Autodesk Fusion 360 part; units mm, degrees
(part 5 of 10)
extrude "Pan blank''''''" add sketch "草图1 (37)" along normal blind 20 separate body makes body 37 in component "Tower_Integrated"
fillet "Outside corner rounds''''''" radius 3 4 edges at (50, 140, 135) (230, 140, 135) (230, 50, 135) (50, 50, 135) on bodies 37 in component "Tower_Integrated"
ref_plane "工作平面2" through (53, 0, 0) normal (1, 0, 0) x (0, 1, 0) in component "Tower_Integrated"
sketch "草图2 (37)" plane through (53, 0, 0) normal (1, 0, 0) x (0, 0, -1) in component "Tower_Integrated"
  line L0 (-135.8318, 53) -> (-129.958, 137)
  line L1 (-129.958, 137) -> (-146, 137)
  line L2 (-146, 137) -> (-146, 53)
  line L3 (-146, 53) -> (-135.8318, 53)
  dimension "d1948" = 135.8318
  dimension "d1950" = 129.958
  dimension "d1952" = 146
  constraint horizontal L1
  constraint vertical L2
  constraint horizontal L3
  measures "d1948" horizontal distance of origin L0.start
  measures "d1950" horizontal distance of origin L0.end
  measures "d1952" horizontal distance of origin L1.end
extrude "Sloped catch cavity''''''" cut sketch "草图2 (37)" along normal blind 174 bodies 37 in component "Tower_Integrated"
ref_plane "工作平面3" through (178, 0, 0) normal (1, 0, 0) x (0, 1, 0) in component "Tower_Integrated"
sketch "草图3 (13)" plane through (178, 0, 0) normal (1, 0, 0) x (0, 0, -1) in component "Tower_Integrated"
  line L0 (-125, 137) -> (-125, 165)
  line L1 (-125, 165) -> (-128, 165)
  line L2 (-128, 165) -> (-129.958, 137)
  line L3 (-129.958, 137) -> (-125, 137)
  dimension "d1960" = 128
  dimension "d1961" = 129.958
  constraint vertical L0
  constraint horizontal L1
  constraint horizontal L3
  measures "d1960" horizontal distance of origin L1.end
  measures "d1961" horizontal distance of origin L2.end
extrude "Drain tongue floor''''''" add sketch "草图3 (13)" along normal blind 34 bodies 37 in component "Tower_Integrated"
ref_plane "工作平面4" through (178, 0, 0) normal (1, 0, 0) x (0, 1, 0) in component "Tower_Integrated"
sketch "草图4 (13)" plane through (178, 0, 0) normal (1, 0, 0) x (0, 0, -1) in component "Tower_Integrated"
  line L0 (-125, 137) -> (-125, 165)
  line L1 (-125, 165) -> (-134, 165)
  line L2 (-134, 165) -> (-135.958, 137)
  line L3 (-135.958, 137) -> (-125, 137)
  dimension "d1969" = 134
  dimension "d1970" = 135.958
  constraint vertical L0
  constraint horizontal L1
  constraint horizontal L3
  measures "d1969" horizontal distance of origin L1.end
  measures "d1970" horizontal distance of origin L2.end
extrude "Tongue side rail''''''" add sketch "草图4 (13)" along normal blind 3 bodies 37 in component "Tower_Integrated"
ref_plane "工作平面5" through (209, 0, 0) normal (1, 0, 0) x (0, 1, 0) in component "Tower_Integrated"
sketch "草图5 (13)" plane through (209, 0, 0) normal (1, 0, 0) x (0, 0, -1) in component "Tower_Integrated"
  line L0 (-125, 137) -> (-125, 165)
  line L1 (-125, 165) -> (-134, 165)
  line L2 (-134, 165) -> (-135.958, 137)
  line L3 (-135.958, 137) -> (-125, 137)
  dimension "d1978" = 134
  dimension "d1979" = 135.958
  constraint vertical L0
  constraint horizontal L1
  constraint horizontal L3
  measures "d1978" horizontal distance of origin L1.end
  measures "d1979" horizontal distance of origin L2.end
extrude "Tongue side rail (1)''''''" add sketch "草图5 (13)" along normal blind 3 bodies 37 in component "Tower_Integrated"
ref_plane "工作平面6" through (181, 0, 0) normal (1, 0, 0) x (0, 1, 0) in component "Tower_Integrated"
sketch "草图6 (13)" plane through (181, 0, 0) normal (1, 0, 0) x (0, 0, -1) in component "Tower_Integrated"
  line L0 (-129.958, 137) -> (-128, 165)
  line L1 (-128, 165) -> (-146, 165)
  line L2 (-146, 165) -> (-146, 137)
  line L3 (-146, 137) -> (-129.958, 137)
  dimension "d1984" = 129.958
  dimension "d1986" = 128
  dimension "d1988" = 146
  constraint horizontal L1
  constraint vertical L2
  constraint horizontal L3
  measures "d1984" horizontal distance of origin L0.start
  measures "d1986" horizontal distance of origin L0.end
  measures "d1988" horizontal distance of origin L1.end
extrude "Open drain mouth''''''" cut sketch "草图6 (13)" along normal blind 28 bodies 37 in component "Tower_Integrated"
ref_plane "工作平面7" through (0, 0, 125) normal (0, 0, 1) x (1, 0, 0) in component "Tower_Integrated"
sketch "草图7 (13)" plane through (0, 0, 125) normal (0, 0, 1) x (1, 0, 0) in component "Tower_Integrated"
  line L0 (53, 53) -> (65, 53)
  line L1 (65, 53) -> (65, 65)
  line L2 (65, 65) -> (53, 65)
  line L3 (53, 65) -> (53, 53)
  dimension "d1995" = 12
  dimension "d1996" = 12
  constraint horizontal L0
  constraint vertical L1
  constraint horizontal L2
  constraint vertical L3
  measures "d1995" horizontal distance of L0.start L0.end
  measures "d1996" vertical distance of L0.end L1.end
extrude "Grate seat 00''''''" add sketch "草图7 (13)" along normal blind 16 bodies 37 in component "Tower_Integrated"
ref_plane "工作平面8" through (0, 0, 125) normal (0, 0, 1) x (1, 0, 0) in component "Tower_Integrated"
sketch "草图8 (13)" plane through (0, 0, 125) normal (0, 0, 1) x (1, 0, 0) in component "Tower_Integrated"
  line L0 (53, 125) -> (65, 125)
  line L1 (65, 125) -> (65, 137)
  line L2 (65, 137) -> (53, 137)
  line L3 (53, 137) -> (53, 125)
  dimension "d2002" = 125
  dimension "d2003" = 12
  dimension "d2004" = 12
  constraint horizontal L0
  constraint vertical L1
  constraint horizontal L2
  constraint vertical L3
  measures "d2002" vertical distance of origin L0.start
  measures "d2003" horizontal distance of L0.start L0.end
  measures "d2004" vertical distance of L0.end L1.end
extrude "Grate seat 01''''''" add sketch "草图8 (13)" along normal blind 16 bodies 37 in component "Tower_Integrated"
ref_plane "工作平面9" through (0, 0, 125) normal (0, 0, 1) x (1, 0, 0) in component "Tower_Integrated"
sketch "草图9 (13)" plane through (0, 0, 125) normal (0, 0, 1) x (1, 0, 0) in component "Tower_Integrated"
  line L0 (215, 53) -> (227, 53)
  line L1 (227, 53) -> (227, 65)
  line L2 (227, 65) -> (215, 65)
  line L3 (215, 65) -> (215, 53)
  dimension "d2009" = 215
  dimension "d2011" = 12
  dimension "d2012" = 12
  constraint horizontal L0
  constraint vertical L1
  constraint horizontal L2
  constraint vertical L3
  measures "d2009" horizontal distance of origin L0.start
  measures "d2011" horizontal distance of L0.start L0.end
  measures "d2012" vertical distance of L0.end L1.end
extrude "Grate seat 10''''''" add sketch "草图9 (13)" along normal blind 16 bodies 37 in component "Tower_Integrated"
ref_plane "工作平面10" through (0, 0, 125) normal (0, 0, 1) x (1, 0, 0) in component "Tower_Integrated"
sketch "草图10 (13)" plane through (0, 0, 125) normal (0, 0, 1) x (1, 0, 0) in component "Tower_Integrated"
  line L0 (215, 125) -> (227, 125)
  line L1 (227, 125) -> (227, 137)
  line L2 (227, 137) -> (215, 137)
  line L3 (215, 137) -> (215, 125)
  dimension "d2017" = 215
  dimension "d2018" = 125
  dimension "d2019" = 12
  dimension "d2020" = 12
  constraint horizontal L0
  constraint vertical L1
  constraint horizontal L2
  constraint vertical L3
  measures "d2017" horizontal distance of origin L0.start
  measures "d2018" vertical distance of origin L0.start
  measures "d2019" horizontal distance of L0.start L0.end
  measures "d2020" vertical distance of L0.end L1.end
extrude "Grate seat 11''''''" add sketch "草图10 (13)" along normal blind 16 bodies 37 in component "Tower_Integrated"
ref_plane "工作平面11" through (178, 0, 0) normal (1, 0, 0) x (0, 1, 0) in component "Tower_Integrated"
sketch "草图11 (13)" plane through (178, 0, 0) normal (1, 0, 0) x (0, 0, -1) in component "Tower_Integrated"
  line L0 (-124.8, 163) -> (-124.8, 164)
  line L1 (-124.8, 164) -> (-125.6, 164)
  line L2 (-125.6, 164) -> (-125.6, 163)
  line L3 (-125.6, 163) -> (-124.8, 163)
  dimension "d2025" = 124.8
  dimension "d2026" = 163
  dimension "d2027" = 164
  dimension "d2028" = 125.6
  constraint vertical L0
  constraint horizontal L1
  constraint vertical L2
  constraint horizontal L3
  measures "d2025" horizontal distance of origin L0.start
  measures "d2026" vertical distance of origin L0.start
  measures "d2027" vertical distance of origin L0.end
  measures "d2028" horizontal distance of origin L1.end
extrude "Drip break underside groove''''''" cut sketch "草图11 (13)" along normal blind 34 bodies 37 in component "Tower_Integrated"
ref_plane "工作平面1" through (0, 0, 141) normal (0, 0, 1) x (1, 0, 0) in component "UP_RemovableGrate"
sketch "草图1 (38)" plane through (0, 0, 141) normal (0, 0, 1) x (1, 0, 0) in component "UP_RemovableGrate"
  line L0 (53.3, 53.3) -> (226.7, 53.3)
  line L1 (226.7, 53.3) -> (226.7, 136.7)
  line L2 (226.7, 136.7) -> (53.3, 136.7)
  line L3 (53.3, 136.7) -> (53.3, 53.3)
  dimension "d2035" = 173.4
  dimension "d2036" = 83.4
  constraint horizontal L0
  constraint vertical L1
  constraint horizontal L2
  constraint vertical L3
  measures "d2035" horizontal distance of L0.start L0.end
  measures "d2036" vertical distance of L0.end L1.end
extrude "Horizontal removable deck''''''" add sketch "草图1 (38)" along normal blind 4 separate body makes body 38 in component "UP_RemovableGrate"
ref_plane "工作平面2" through (0, 0, 141) normal (0, 0, 1) x (1, 0, 0) in component "UP_RemovableGrate"
sketch "草图2 (38)" plane through (0, 0, 141) normal (0, 0, 1) x (1, 0, 0) in component "UP_RemovableGrate"
  line L0 (68, 60.3) -> (72, 60.3)
  line L1 (72, 60.3) -> (72, 129.7)
  line L2 (72, 129.7) -> (68, 129.7)
  line L3 (68, 129.7) -> (68, 60.3)
  dimension "d2041" = 68
  dimension "d2043" = 4
  dimension "d2044" = 69.4
  constraint horizontal L0
  constraint vertical L1
  constraint horizontal L2
  constraint vertical L3
  measures "d2041" horizontal distance of origin L0.start
  measures "d2043" horizontal distance of L0.start L0.end
  measures "d2044" vertical distance of L0.end L1.end
extrude "Drain slot 1''''''" cut sketch "草图2 (38)" along normal blind 4 bodies 38 in component "UP_RemovableGrate"
ref_plane "工作平面3" through (0, 0, 141) normal (0, 0, 1) x (1, 0, 0) in component "UP_RemovableGrate"
sketch "草图3 (14)" plane through (0, 0, 141) normal (0, 0, 1) x (1, 0, 0) in component "UP_RemovableGrate"
  line L0 (78, 60.3) -> (82, 60.3)
  line L1 (82, 60.3) -> (82, 129.7)
  line L2 (82, 129.7) -> (78, 129.7)
  line L3 (78, 129.7) -> (78, 60.3)
  dimension "d2049" = 78
  dimension "d2051" = 4
  dimension "d2052" = 69.4
  constraint horizontal L0
  constraint vertical L1
  constraint horizontal L2
  constraint vertical L3
  measures "d2049" horizontal distance of origin L0.start
  measures "d2051" horizontal distance of L0.start L0.end
  measures "d2052" vertical distance of L0.end L1.end
extrude "Drain slot 2''''''" cut sketch "草图3 (14)" along normal blind 4 bodies 38 in component "UP_RemovableGrate"
ref_plane "工作平面4" through (0, 0, 141) normal (0, 0, 1) x (1, 0, 0) in component "UP_RemovableGrate"
sketch "草图4 (14)" plane through (0, 0, 141) normal (0, 0, 1) x (1, 0, 0) in component "UP_RemovableGrate"
  line L0 (88, 60.3) -> (92, 60.3)
  line L1 (92, 60.3) -> (92, 129.7)
  line L2 (92, 129.7) -> (88, 129.7)
  line L3 (88, 129.7) -> (88, 60.3)
  dimension "d2057" = 88
  dimension "d2059" = 4
  dimension "d2060" = 69.4
  constraint horizontal L0
  constraint vertical L1
  constraint horizontal L2
  constraint vertical L3
  measures "d2057" horizontal distance of origin L0.start
  measures "d2059" horizontal distance of L0.start L0.end
  measures "d2060" vertical distance of L0.end L1.end
extrude "Drain slot 3''''''" cut sketch "草图4 (14)" along normal blind 4 bodies 38 in component "UP_RemovableGrate"
ref_plane "工作平面5" through (0, 0, 141) normal (0, 0, 1) x (1, 0, 0) in component "UP_RemovableGrate"
sketch "草图5 (14)" plane through (0, 0, 141) normal (0, 0, 1) x (1, 0, 0) in component "UP_RemovableGrate"
  line L0 (98, 60.3) -> (102, 60.3)
  line L1 (102, 60.3) -> (102, 129.7)
  line L2 (102, 129.7) -> (98, 129.7)
  line L3 (98, 129.7) -> (98, 60.3)
  dimension "d2065" = 98
  dimension "d2067" = 4
  dimension "d2068" = 69.4
  constraint horizontal L0
  constraint vertical L1
  constraint horizontal L2
  constraint vertical L3
  measures "d2065" horizontal distance of origin L0.start
  measures "d2067" horizontal distance of L0.start L0.end
  measures "d2068" vertical distance of L0.end L1.end
extrude "Drain slot 4''''''" cut sketch "草图5 (14)" along normal blind 4 bodies 38 in component "UP_RemovableGrate"
ref_plane "工作平面6" through (0, 0, 141) normal (0, 0, 1) x (1, 0, 0) in component "UP_RemovableGrate"
sketch "草图6 (14)" plane through (0, 0, 141) normal (0, 0, 1) x (1, 0, 0) in component "UP_RemovableGrate"
  line L0 (108, 60.3) -> (112, 60.3)
  line L1 (112, 60.3) -> (112, 129.7)
  line L2 (112, 129.7) -> (108, 129.7)
  line L3 (108, 129.7) -> (108, 60.3)
  dimension "d2073" = 108
  dimension "d2075" = 4
  dimension "d2076" = 69.4
  constraint horizontal L0
  constraint vertical L1
  constraint horizontal L2
  constraint vertical L3
  measures "d2073" horizontal distance of origin L0.start
  measures "d2075" horizontal distance of L0.start L0.end
  measures "d2076" vertical distance of L0.end L1.end
extrude "Drain slot 5''''''" cut sketch "草图6 (14)" along normal blind 4 bodies 38 in component "UP_RemovableGrate"
ref_plane "工作平面7" through (0, 0, 141) normal (0, 0, 1) x (1, 0, 0) in component "UP_RemovableGrate"
sketch "草图7 (14)" plane through (0, 0, 141) normal (0, 0, 1) x (1, 0, 0) in component "UP_RemovableGrate"
  line L0 (118, 60.3) -> (122, 60.3)
  line L1 (122, 60.3) -> (122, 129.7)
  line L2 (122, 129.7) -> (118, 129.7)
  line L3 (118, 129.7) -> (118, 60.3)
  dimension "d2081" = 118
  dimension "d2083" = 4
  dimension "d2084" = 69.4
  constraint horizontal L0
  constraint vertical L1
  constraint horizontal L2
  constraint vertical L3
  measures "d2081" horizontal distance of origin L0.start
  measures "d2083" horizontal distance of L0.start L0.end
  measures "d2084" vertical distance of L0.end L1.end
extrude "Drain slot 6''''''" cut sketch "草图7 (14)" along normal blind 4 bodies 38 in component "UP_RemovableGrate"
ref_plane "工作平面8" through (0, 0, 141) normal (0, 0, 1) x (1, 0, 0) in component "UP_RemovableGrate"
sketch "草图8 (14)" plane through (0, 0, 141) normal (0, 0, 1) x (1, 0, 0) in component "UP_RemovableGrate"
  line L0 (128, 60.3) -> (132, 60.3)
  line L1 (132, 60.3) -> (132, 129.7)
  line L2 (132, 129.7) -> (128, 129.7)
  line L3 (128, 129.7) -> (128, 60.3)
  dimension "d2089" = 128
  dimension "d2091" = 4
  dimension "d2092" = 69.4
  constraint horizontal L0
  constraint vertical L1
  constraint horizontal L2
  constraint vertical L3
  measures "d2089" horizontal distance of origin L0.start
  measures "d2091" horizontal distance of L0.start L0.end
  measures "d2092" vertical distance of L0.end L1.end
extrude "Drain slot 7''''''" cut sketch "草图8 (14)" along normal blind 4 bodies 38 in component "UP_RemovableGrate"
ref_plane "工作平面9" through (0, 0, 141) normal (0, 0, 1) x (1, 0, 0) in component "UP_RemovableGrate"
sketch "草图9 (14)" plane through (0, 0, 141) normal (0, 0, 1) x (1, 0, 0) in component "UP_RemovableGrate"
  line L0 (138, 60.3) -> (142, 60.3)
  line L1 (142, 60.3) -> (142, 129.7)
  line L2 (142, 129.7) -> (138, 129.7)
  line L3 (138, 129.7) -> (138, 60.3)
  dimension "d2097" = 138
  dimension "d2099" = 4
  dimension "d2100" = 69.4
  constraint horizontal L0
  constraint vertical L1
  constraint horizontal L2
  constraint vertical L3
  measures "d2097" horizontal distance of origin L0.start
  measures "d2099" horizontal distance of L0.start L0.end
  measures "d2100" vertical distance of L0.end L1.end
extrude "Drain slot 8''''''" cut sketch "草图9 (14)" along normal blind 4 bodies 38 in component "UP_RemovableGrate"
ref_plane "工作平面10" through (0, 0, 141) normal (0, 0, 1) x (1, 0, 0) in component "UP_RemovableGrate"
sketch "草图10 (14)" plane through (0, 0, 141) normal (0, 0, 1) x (1, 0, 0) in component "UP_RemovableGrate"
  line L0 (148, 60.3) -> (152, 60.3)
  line L1 (152, 60.3) -> (152, 129.7)
  line L2 (152, 129.7) -> (148, 129.7)
  line L3 (148, 129.7) -> (148, 60.3)
  dimension "d2105" = 148
  dimension "d2107" = 4
  dimension "d2108" = 69.4
  constraint horizontal L0
  constraint vertical L1
  constraint horizontal L2
  constraint vertical L3
  measures "d2105" horizontal distance of origin L0.start
  measures "d2107" horizontal distance of L0.start L0.end
  measures "d2108" vertical distance of L0.end L1.end
extrude "Drain slot 9''''''" cut sketch "草图10 (14)" along normal blind 4 bodies 38 in component "UP_RemovableGrate"
ref_plane "工作平面11" through (0, 0, 141) normal (0, 0, 1) x (1, 0, 0) in component "UP_RemovableGrate"
sketch "草图11 (14)" plane through (0, 0, 141) normal (0, 0, 1) x (1, 0, 0) in component "UP_RemovableGrate"
  line L0 (158, 60.3) -> (162, 60.3)
  line L1 (162, 60.3) -> (162, 129.7)
  line L2 (162, 129.7) -> (158, 129.7)
  line L3 (158, 129.7) -> (158, 60.3)
  dimension "d2113" = 158
  dimension "d2115" = 4
  dimension "d2116" = 69.4
  constraint horizontal L0
  constraint vertical L1
  constraint horizontal L2
  constraint vertical L3
  measures "d2113" horizontal distance of origin L0.start
  measures "d2115" horizontal distance of L0.start L0.end
  measures "d2116" vertical distance of L0.end L1.end
extrude "Drain slot 10''''''" cut sketch "草图11 (14)" along normal blind 4 bodies 38 in component "UP_RemovableGrate"
ref_plane "工作平面12" through (0, 0, 141) normal (0, 0, 1) x (1, 0, 0) in component "UP_RemovableGrate"
sketch "草图12 (13)" plane through (0, 0, 141) normal (0, 0, 1) x (1, 0, 0) in component "UP_RemovableGrate"
  line L0 (168, 60.3) -> (172, 60.3)
  line L1 (172, 60.3) -> (172, 129.7)
  line L2 (172, 129.7) -> (168, 129.7)
  line L3 (168, 129.7) -> (168, 60.3)
  dimension "d2121" = 168
  dimension "d2123" = 4
  dimension "d2124" = 69.4
  constraint horizontal L0
  constraint vertical L1
  constraint horizontal L2
  constraint vertical L3
  measures "d2121" horizontal distance of origin L0.start
  measures "d2123" horizontal distance of L0.start L0.end
  measures "d2124" vertical distance of L0.end L1.end
extrude "Drain slot 11''''''" cut sketch "草图12 (13)" along normal blind 4 bodies 38 in component "UP_RemovableGrate"
ref_plane "工作平面13" through (0, 0, 141) normal (0, 0, 1) x (1, 0, 0) in component "UP_RemovableGrate"
sketch "草图13 (13)" plane through (0, 0, 141) normal (0, 0, 1) x (1, 0, 0) in component "UP_RemovableGrate"
  line L0 (178, 60.3) -> (182, 60.3)
  line L1 (182, 60.3) -> (182, 129.7)
  line L2 (182, 129.7) -> (178, 129.7)
  line L3 (178, 129.7) -> (178, 60.3)
  dimension "d2129" = 178
  dimension "d2131" = 4
  dimension "d2132" = 69.4
  constraint horizontal L0
  constraint vertical L1
  constraint horizontal L2
  constraint vertical L3
  measures "d2129" horizontal distance of origin L0.start
  measures "d2131" horizontal distance of L0.start L0.end
  measures "d2132" vertical distance of L0.end L1.end
extrude "Drain slot 12''''" cut sketch "草图13 (13)" along normal blind 4 bodies 38 in component "UP_RemovableGrate"
ref_plane "工作平面14" through (0, 0, 141) normal (0, 0, 1) x (1, 0, 0) in component "UP_RemovableGrate"
sketch "草图14 (11)" plane through (0, 0, 141) normal (0, 0, 1) x (1, 0, 0) in component "UP_RemovableGrate"
  line L0 (188, 60.3) -> (192, 60.3)
  line L1 (192, 60.3) -> (192, 129.7)
  line L2 (192, 129.7) -> (188, 129.7)
  line L3 (188, 129.7) -> (188, 60.3)
  dimension "d2137" = 188
  dimension "d2139" = 4
  dimension "d2140" = 69.4
  constraint horizontal L0
  constraint vertical L1
  constraint horizontal L2
  constraint vertical L3
  measures "d2137" horizontal distance of origin L0.start
  measures "d2139" horizontal distance of L0.start L0.end
  measures "d2140" vertical distance of L0.end L1.end
extrude "Drain slot 13''''" cut sketch "草图14 (11)" along normal blind 4 bodies 38 in component "UP_RemovableGrate"
ref_plane "工作平面15" through (0, 0, 141) normal (0, 0, 1) x (1, 0, 0) in component "UP_RemovableGrate"
sketch "草图15 (11)" plane through (0, 0, 141) normal (0, 0, 1) x (1, 0, 0) in component "UP_RemovableGrate"
  line L0 (198, 60.3) -> (202, 60.3)
  line L1 (202, 60.3) -> (202, 129.7)
  line L2 (202, 129.7) -> (198, 129.7)
  line L3 (198, 129.7) -> (198, 60.3)
  dimension "d2145" = 198
  dimension "d2147" = 4
  dimension "d2148" = 69.4
  constraint horizontal L0
  constraint vertical L1
  constraint horizontal L2
  constraint vertical L3
  measures "d2145" horizontal distance of origin L0.start
  measures "d2147" horizontal distance of L0.start L0.end
  measures "d2148" vertical distance of L0.end L1.end
extrude "Drain slot 14'''" cut sketch "草图15 (11)" along normal blind 4 bodies 38 in component "UP_RemovableGrate"
ref_plane "工作平面16" through (0, 0, 141) normal (0, 0, 1) x (1, 0, 0) in component "UP_RemovableGrate"
sketch "草图16 (4)" plane through (0, 0, 141) normal (0, 0, 1) x (1, 0, 0) in component "UP_RemovableGrate"
  line L0 (208, 60.3) -> (212, 60.3)
  line L1 (212, 60.3) -> (212, 129.7)
  line L2 (212, 129.7) -> (208, 129.7)
  line L3 (208, 129.7) -> (208, 60.3)
  dimension "d2153" = 208
  dimension "d2155" = 4
  dimension "d2156" = 69.4
  constraint horizontal L0
  constraint vertical L1
  constraint horizontal L2
  constraint vertical L3
  measures "d2153" horizontal distance of origin L0.start
  measures "d2155" horizontal distance of L0.start L0.end
  measures "d2156" vertical distance of L0.end L1.end
extrude "Drain slot 15'''" cut sketch "草图16 (4)" along normal blind 4 bodies 38 in component "UP_RemovableGrate"
ref_plane "工作平面17" through (0, 0, 141) normal (0, 0, 1) x (1, 0, 0) in component "UP_RemovableGrate"
sketch "草图17 (4)" plane through (0, 0, 141) normal (0, 0, 1) x (1, 0, 0) in component "UP_RemovableGrate"
  line L0 (132, 132.7) -> (148, 132.7)
  line L1 (148, 132.7) -> (148, 137.7)
  line L2 (148, 137.7) -> (132, 137.7)
  line L3 (132, 137.7) -> (132, 132.7)
  dimension "d2161" = 132
  dimension "d2162" = 132.7
  dimension "d2163" = 16
  dimension "d2164" = 5
  constraint horizontal L0
  constraint vertical L1
  constraint horizontal L2
  constraint vertical L3
  measures "d2161" horizontal distance of origin L0.start
  measures "d2162" vertical distance of origin L0.start
  measures "d2163" horizontal distance of L0.start L0.end
  measures "d2164" vertical distance of L0.end L1.end
extrude "Finger lift notch''''''" cut sketch "草图17 (4)" along normal blind 4 bodies 38 in component "UP_RemovableGrate"
ref_plane "工作平面1" through (0, 0, 0) normal (0, 0, 1) x (1, 0, 0) in component "Tower_SideFrame_1"
sketch "草图1 (39)" plane through (0, 0, 0) normal (0, 0, 1) x (1, 0, 0) in component "Tower_SideFrame_1"
  line L0 (50, 50) -> (58, 50)
  line L1 (58, 50) -> (58, 140)
  line L2 (58, 140) -> (50, 140)
  line L3 (50, 140) -> (50, 50)
  dimension "d2169" = 50
  dimension "d2170" = 50
  dimension "d2171" = 8
  dimension "d2172" = 90
  constraint horizontal L0
  constraint vertical L1
  constraint horizontal L2
  constraint vertical L3
  measures "d2169" horizontal distance of origin L0.start
  measures "d2170" vertical distance of origin L0.start
  measures "d2171" horizontal distance of L0.start L0.end
  measures "d2172" vertical distance of L0.end L1.end
extrude "Portal frame blank" add sketch "草图1 (39)" along normal blind 125 separate body makes body 39 in component "Tower_SideFrame_1"
ref_plane "工作平面2" through (50, 0, 0) normal (1, 0, 0) x (0, 1, 0) in component "Tower_SideFrame_1"
sketch "草图2 (39)" plane through (50, 0, 0) normal (1, 0, 0) x (0, 0, -1) in component "Tower_SideFrame_1"
  line L0 (-8, 62) -> (-8, 128)
  line L1 (-8, 128) -> (-117, 128)
  line L2 (-117, 128) -> (-117, 62)
  line L3 (-117, 62) -> (-8, 62)
  dimension "d2177" = 8
  dimension "d2178" = 62
  dimension "d2179" = 128
  dimension "d2180" = 117
  constraint vertical L0
  constraint horizontal L1
  constraint vertical L2
  constraint horizontal L3
  measures "d2177" horizontal distance of origin L0.start
  measures "d2178" vertical distance of origin L0.start
  measures "d2179" vertical distance of origin L0.end
  measures "d2180" horizontal distance of origin L1.end
extrude "Open portal" cut sketch "草图2 (39)" along normal blind 8 bodies 39 in component "Tower_SideFrame_1"
ref_plane "工作平面3" through (0, 0, 125) normal (0, 0, 1) x (1, 0, 0) in component "Tower_SideFrame_1"
sketch "草图3 (15)" plane through (0, 0, 125) normal (0, 0, 1) x (1, 0, 0) in component "Tower_SideFrame_1"
  line L0 (51.5, 55.5) -> (56.5, 55.5)
  line L1 (56.5, 55.5) -> (56.5, 60.5)
  line L2 (56.5, 60.5) -> (51.5, 60.5)
  line L3 (51.5, 60.5) -> (51.5, 55.5)
  dimension "d2185" = 51.5
  dimension "d2186" = 55.5
  dimension "d2187" = 5
  dimension "d2188" = 5
  constraint horizontal L0
  constraint vertical L1
  constraint horizontal L2
  constraint vertical L3
  measures "d2185" horizontal distance of origin L0.start
  measures "d2186" vertical distance of origin L0.start
  measures "d2187" horizontal distance of L0.start L0.end
  measures "d2188" vertical distance of L0.end L1.end
extrude "Upper tray locating key" add sketch "草图3 (15)" along normal blind 1.5 bodies 39 in component "Tower_SideFrame_1"
ref_plane "工作平面4" through (0, 0, 125) normal (0, 0, 1) x (1, 0, 0) in component "Tower_SideFrame_1"
sketch "草图4 (15)" plane through (0, 0, 125) normal (0, 0, 1) x (1, 0, 0) in component "Tower_SideFrame_1"
  line L0 (51.5, 129.5) -> (56.5, 129.5)
  line L1 (56.5, 129.5) -> (56.5, 134.5)
  line L2 (56.5, 134.5) -> (51.5, 134.5)
  line L3 (51.5, 134.5) -> (51.5, 129.5)
  dimension "d2193" = 51.5
  dimension "d2194" = 129.5
  dimension "d2195" = 5
  dimension "d2196" = 5
  constraint horizontal L0
  constraint vertical L1
  constraint horizontal L2
  constraint vertical L3
  measures "d2193" horizontal distance of origin L0.start
  measures "d2194" vertical distance of origin L0.start
  measures "d2195" horizontal distance of L0.start L0.end
  measures "d2196" vertical distance of L0.end L1.end
extrude "Upper tray locating key (1)" add sketch "草图4 (15)" along normal blind 1.5 bodies 39 in component "Tower_SideFrame_1"
ref_plane "工作平面1" through (0, 0, 0) normal (0, 0, 1) x (1, 0, 0) in component "Tower_SideFrame_2"
sketch "草图1 (40)" plane through (0, 0, 0) normal (0, 0, 1) x (1, 0, 0) in component "Tower_SideFrame_2"
  line L0 (222, 50) -> (230, 50)
  line L1 (230, 50) -> (230, 140)
  line L2 (230, 140) -> (222, 140)
  line L3 (222, 140) -> (222, 50)
  dimension "d2201" = 222
  dimension "d2202" = 50
  dimension "d2203" = 8
  dimension "d2204" = 90
  constraint horizontal L0
  constraint vertical L1
  constraint horizontal L2
  constraint vertical L3
  measures "d2201" horizontal distance of origin L0.start
  measures "d2202" vertical distance of origin L0.start
  measures "d2203" horizontal distance of L0.start L0.end
  measures "d2204" vertical distance of L0.end L1.end
extrude "Portal frame blank'" add sketch "草图1 (40)" along normal blind 125 separate body makes body 40 in component "Tower_SideFrame_2"
ref_plane "工作平面2" through (222, 0, 0) normal (1, 0, 0) x (0, 1, 0) in component "Tower_SideFrame_2"
sketch "草图2 (40)" plane through (222, 0, 0) normal (1, 0, 0) x (0, 0, -1) in component "Tower_SideFrame_2"
  line L0 (-8, 62) -> (-8, 128)
  line L1 (-8, 128) -> (-117, 128)
  line L2 (-117, 128) -> (-117, 62)
  line L3 (-117, 62) -> (-8, 62)
  dimension "d2209" = 8
  dimension "d2210" = 62
  dimension "d2211" = 128
  dimension "d2212" = 117
  constraint vertical L0
  constraint horizontal L1
  constraint vertical L2
  constraint horizontal L3
  measures "d2209" horizontal distance of origin L0.start
  measures "d2210" vertical distance of origin L0.start
  measures "d2211" vertical distance of origin L0.end
  measures "d2212" horizontal distance of origin L1.end
extrude "Open portal'" cut sketch "草图2 (40)" along normal blind 8 bodies 40 in component "Tower_SideFrame_2"
ref_plane "工作平面3" through (0, 0, 125) normal (0, 0, 1) x (1, 0, 0) in component "Tower_SideFrame_2"
sketch "草图3 (16)" plane through (0, 0, 125) normal (0, 0, 1) x (1, 0, 0) in component "Tower_SideFrame_2"
  line L0 (223.5, 55.5) -> (228.5, 55.5)
  line L1 (228.5, 55.5) -> (228.5, 60.5)
  line L2 (228.5, 60.5) -> (223.5, 60.5)
  line L3 (223.5, 60.5) -> (223.5, 55.5)
  dimension "d2217" = 223.5
  dimension "d2218" = 55.5
  dimension "d2219" = 5
  dimension "d2220" = 5
  constraint horizontal L0
  constraint vertical L1
  constraint horizontal L2
  constraint vertical L3
  measures "d2217" horizontal distance of origin L0.start
  measures "d2218" vertical distance of origin L0.start
  measures "d2219" horizontal distance of L0.start L0.end
  measures "d2220" vertical distance of L0.end L1.end
extrude "Upper tray locating key'" add sketch "草图3 (16)" along normal blind 1.5 bodies 40 in component "Tower_SideFrame_2"
ref_plane "工作平面4" through (0, 0, 125) normal (0, 0, 1) x (1, 0, 0) in component "Tower_SideFrame_2"
sketch "草图4 (16)" plane through (0, 0, 125) normal (0, 0, 1) x (1, 0, 0) in component "Tower_SideFrame_2"
  line L0 (223.5, 129.5) -> (228.5, 129.5)
  line L1 (228.5, 129.5) -> (228.5, 134.5)
  line L2 (228.5, 134.5) -> (223.5, 134.5)
  line L3 (223.5, 134.5) -> (223.5, 129.5)
  dimension "d2225" = 223.5
  dimension "d2226" = 129.5
  dimension "d2227" = 5
  dimension "d2228" = 5
  constraint horizontal L0
  constraint vertical L1
  constraint horizontal L2
  constraint vertical L3
  measures "d2225" horizontal distance of origin L0.start
  measures "d2226" vertical distance of origin L0.start
  measures "d2227" horizontal distance of L0.start L0.end
  measures "d2228" vertical distance of L0.end L1.end
extrude "Upper tray locating key (1)'" add sketch "草图4 (16)" along normal blind 1.5 bodies 40 in component "Tower_SideFrame_2"
ref_plane "工作平面12" through (0, 0, 125) normal (0, 0, 1) x (1, 0, 0) in component "Tower_Integrated"
sketch "草图12 (14)" plane through (0, 0, 125) normal (0, 0, 1) x (1, 0, 0) in component "Tower_Integrated"
  line L0 (51.25, 55.25) -> (56.75, 55.25)
  line L1 (56.75, 55.25) -> (56.75, 60.75)
  line L2 (56.75, 60.75) -> (51.25, 60.75)
  line L3 (51.25, 60.75) -> (51.25, 55.25)
  dimension "d2233" = 51.25
  dimension "d2234" = 55.25
  dimension "d2235" = 5.5
  dimension "d2236" = 5.5
  constraint horizontal L0
  constraint vertical L1
  constraint horizontal L2
  constraint vertical L3
  measures "d2233" horizontal distance of origin L0.start
  measures "d2234" vertical distance of origin L0.start
  measures "d2235" horizontal distance of L0.start L0.end
  measures "d2236" vertical distance of L0.end L1.end
extrude "Upper frame key socket" cut sketch "草图12 (14)" along normal blind 1.8 bodies 37 in component "Tower_Integrated"
ref_plane "工作平面13" through (0, 0, 125) normal (0, 0, 1) x (1, 0, 0) in component "Tower_Integrated"
sketch "草图13 (14)" plane through (0, 0, 125) normal (0, 0, 1) x (1, 0, 0) in component "Tower_Integrated"
  line L0 (51.25, 129.25) -> (56.75, 129.25)
  line L1 (56.75, 129.25) -> (56.75, 134.75)
  line L2 (56.75, 134.75) -> (51.25, 134.75)
  line L3 (51.25, 134.75) -> (51.25, 129.25)
  dimension "d2241" = 51.25
  dimension "d2242" = 129.25
  dimension "d2243" = 5.5
  dimension "d2244" = 5.5
  constraint horizontal L0
  constraint vertical L1
  constraint horizontal L2
  constraint vertical L3
  measures "d2241" horizontal distance of origin L0.start
  measures "d2242" vertical distance of origin L0.start
  measures "d2243" horizontal distance of L0.start L0.end
  measures "d2244" vertical distance of L0.end L1.end
extrude "Upper frame key socket (1)" cut sketch "草图13 (14)" along normal blind 1.8 bodies 37 in component "Tower_Integrated"
ref_plane "工作平面14" through (0, 0, 125) normal (0, 0, 1) x (1, 0, 0) in component "Tower_Integrated"
sketch "草图14 (12)" plane through (0, 0, 125) normal (0, 0, 1) x (1, 0, 0) in component "Tower_Integrated"
  line L0 (223.25, 55.25) -> (228.75, 55.25)
  line L1 (228.75, 55.25) -> (228.75, 60.75)
  line L2 (228.75, 60.75) -> (223.25, 60.75)
  line L3 (223.25, 60.75) -> (223.25, 55.25)
  dimension "d2249" = 223.25
  dimension "d2250" = 55.25
  dimension "d2251" = 5.5
  dimension "d2252" = 5.5
  constraint horizontal L0
  constraint vertical L1
  constraint horizontal L2
  constraint vertical L3
  measures "d2249" horizontal distance of origin L0.start
  measures "d2250" vertical distance of origin L0.start
  measures "d2251" horizontal distance of L0.start L0.end
  measures "d2252" vertical distance of L0.end L1.end
extrude "Upper frame key socket (2)" cut sketch "草图14 (12)" along normal blind 1.8 bodies 37 in component "Tower_Integrated"
ref_plane "工作平面15" through (0, 0, 125) normal (0, 0, 1) x (1, 0, 0) in component "Tower_Integrated"
sketch "草图15 (12)" plane through (0, 0, 125) normal (0, 0, 1) x (1, 0, 0) in component "Tower_Integrated"
  line L0 (223.25, 129.25) -> (228.75, 129.25)
  line L1 (228.75, 129.25) -> (228.75, 134.75)
  line L2 (228.75, 134.75) -> (223.25, 134.75)
  line L3 (223.25, 134.75) -> (223.25, 129.25)
  dimension "d2257" = 223.25
  dimension "d2258" = 129.25
  dimension "d2259" = 5.5
  dimension "d2260" = 5.5
  constraint horizontal L0
  constraint vertical L1
  constraint horizontal L2
  constraint vertical L3
  measures "d2257" horizontal distance of origin L0.start
  measures "d2258" vertical distance of origin L0.start
  measures "d2259" horizontal distance of L0.start L0.end
  measures "d2260" vertical distance of L0.end L1.end
extrude "Upper frame key socket (3)" cut sketch "草图15 (12)" along normal blind 1.8 bodies 37 in component "Tower_Integrated"
ref_plane "工作平面1" through (0, 0, 0) normal (0, 0, 1) x (1, 0, 0) in component "FIT_Tight"
sketch "草图1 (41)" plane through (0, 0, 0) normal (0, 0, 1) x (1, 0, 0) in component "FIT_Tight"
  line L0 (880, 50) -> (904, 50)
  line L1 (904, 50) -> (904, 74)
  line L2 (904, 74) -> (880, 74)
  line L3 (880, 74) -> (880, 50)
  dimension "d2265" = 880
  dimension "d2266" = 50
  dimension "d2267" = 24
  dimension "d2268" = 24
  constraint horizontal L0
  constraint vertical L1
  constraint horizontal L2
  constraint vertical L3
  measures "d2265" horizontal distance of origin L0.start
  measures "d2266" vertical distance of origin L0.start
  measures "d2267" horizontal distance of L0.start L0.end
  measures "d2268" vertical distance of L0.end L1.end
extrude "Fit coupon plate" add sketch "草图1 (41)" along normal blind 4 separate body makes body 41 in component "FIT_Tight"
ref_plane "工作平面2" through (0, 0, 0) normal (0, 0, 1) x (1, 0, 0) in component "FIT_Tight"
sketch "草图2 (41)" plane through (0, 0, 0) normal (0, 0, 1) x (1, 0, 0) in component "FIT_Tight"
  line L0 (887.8, 57.8) -> (896.2, 57.8)
  line L1 (896.2, 57.8) -> (896.2, 66.2)
  line L2 (896.2, 66.2) -> (887.8, 66.2)
  line L3 (887.8, 66.2) -> (887.8, 57.8)
  dimension "d2273" = 887.8
  dimension "d2274" = 57.8
  dimension "d2275" = 8.4
  dimension "d2276" = 8.4
  constraint horizontal L0
  constraint vertical L1
  constraint horizontal L2
  constraint vertical L3
  measures "d2273" horizontal distance of origin L0.start
  measures "d2274" vertical distance of origin L0.start
  measures "d2275" horizontal distance of L0.start L0.end
  measures "d2276" vertical distance of L0.end L1.end
extrude "Foot locating socket" cut sketch "草图2 (41)" along normal blind 1.8 bodies 41 in component "FIT_Tight"
ref_plane "工作平面1" through (0, 0, 0) normal (0, 0, 1) x (1, 0, 0) in component "FIT_Nominal"
sketch "草图1 (42)" plane through (0, 0, 0) normal (0, 0, 1) x (1, 0, 0) in component "FIT_Nominal"
  line L0 (910, 50) -> (934, 50)
  line L1 (934, 50) -> (934, 74)
  line L2 (934, 74) -> (910, 74)
  line L3 (910, 74) -> (910, 50)
  dimension "d2281" = 910
  dimension "d2282" = 50
  dimension "d2283" = 24
  dimension "d2284" = 24
  constraint horizontal L0
  constraint vertical L1
  constraint horizontal L2
  constraint vertical L3
  measures "d2281" horizontal distance of origin L0.start
  measures "d2282" vertical distance of origin L0.start
  measures "d2283" horizontal distance of L0.start L0.end
  measures "d2284" vertical distance of L0.end L1.end
extrude "Fit coupon plate'" add sketch "草图1 (42)" along normal blind 4 separate body makes body 42 in component "FIT_Nominal"
ref_plane "工作平面2" through (0, 0, 0) normal (0, 0, 1) x (1, 0, 0) in component "FIT_Nominal"
sketch "草图2 (42)" plane through (0, 0, 0) normal (0, 0, 1) x (1, 0, 0) in component "FIT_Nominal"
  line L0 (917.75, 57.75) -> (926.25, 57.75)
  line L1 (926.25, 57.75) -> (926.25, 66.25)
  line L2 (926.25, 66.25) -> (917.75, 66.25)
  line L3 (917.75, 66.25) -> (917.75, 57.75)
  dimension "d2289" = 917.75
  dimension "d2290" = 57.75
  dimension "d2291" = 8.5
  dimension "d2292" = 8.5
  constraint horizontal L0
  constraint vertical L1
  constraint horizontal L2
  constraint vertical L3
  measures "d2289" horizontal distance of origin L0.start
  measures "d2290" vertical distance of origin L0.start
  measures "d2291" horizontal distance of L0.start L0.end
  measures "d2292" vertical distance of L0.end L1.end
extrude "Foot locating socket'" cut sketch "草图2 (42)" along normal blind 1.8 bodies 42 in component "FIT_Nominal"
ref_plane "工作平面1" through (0, 0, 0) normal (0, 0, 1) x (1, 0, 0) in component "FIT_Loose"
sketch "草图1 (43)" plane through (0, 0, 0) normal (0, 0, 1) x (1, 0, 0) in component "FIT_Loose"
  line L0 (940, 50) -> (964, 50)
  line L1 (964, 50) -> (964, 74)
  line L2 (964, 74) -> (940, 74)
  line L3 (940, 74) -> (940, 50)
  dimension "d2297" = 940
  dimension "d2298" = 50
  dimension "d2299" = 24
  dimension "d2300" = 24
  constraint horizontal L0
  constraint vertical L1
  constraint horizontal L2
  constraint vertical L3
  measures "d2297" horizontal distance of origin L0.start
  measures "d2298" vertical distance of origin L0.start
  measures "d2299" horizontal distance of L0.start L0.end
  measures "d2300" vertical distance of L0.end L1.end
extrude "Fit coupon plate''" add sketch "草图1 (43)" along normal blind 4 separate body makes body 43 in component "FIT_Loose"
ref_plane "工作平面2" through (0, 0, 0) normal (0, 0, 1) x (1, 0, 0) in component "FIT_Loose"
sketch "草图2 (43)" plane through (0, 0, 0) normal (0, 0, 1) x (1, 0, 0) in component "FIT_Loose"
  line L0 (947.7, 57.7) -> (956.3, 57.7)
  line L1 (956.3, 57.7) -> (956.3, 66.3)
  line L2 (956.3, 66.3) -> (947.7, 66.3)
  line L3 (947.7, 66.3) -> (947.7, 57.7)
  dimension "d2305" = 947.7
  dimension "d2306" = 57.7
  dimension "d2307" = 8.6
  dimension "d2308" = 8.6
  constraint horizontal L0
  constraint vertical L1
  constraint horizontal L2
  constraint vertical L3
  measures "d2305" horizontal distance of origin L0.start
  measures "d2306" vertical distance of origin L0.start
  measures "d2307" horizontal distance of L0.start L0.end
  measures "d2308" vertical distance of L0.end L1.end
extrude "Foot locating socket''" cut sketch "草图2 (43)" along normal blind 1.8 bodies 43 in component "FIT_Loose"
ref_plane "工作平面16" through (0, 0, 19.8) normal (0, 0, 1) x (1, 0, 0) in component "L1_DrainPan"
sketch "草图16 (5)" plane through (0, 0, 19.8) normal (0, 0, 1) x (1, 0, 0) in component "L1_DrainPan"
  line L0 (59, 140) -> (221, 140)
  line L1 (221, 140) -> (221, 167)
  line L2 (221, 167) -> (59, 167)
  line L3 (59, 167) -> (59, 140)
  dimension "d2314" = 59
  dimension "d2316" = 162
  dimension "d2317" = 27
  constraint horizontal L0
  constraint vertical L1
  constraint horizontal L2
  constraint vertical L3
  measures "d2314" horizontal distance of origin L0.start
  measures "d2316" horizontal distance of L0.start L0.end
  measures "d2317" vertical distance of L0.end L1.end
extrude "R02 remove projecting spout" cut sketch "草图16 (5)" along normal blind 20.4 bodies 1 in component "L1_DrainPan"
ref_plane "工作平面17" through (63, 0, 0) normal (1, 0, 0) x (0, 1, 0) in component "L1_DrainPan"
sketch "草图17 (5)" plane through (63, 0, 0) normal (1, 0, 0) x (0, 0, -1) in component "L1_DrainPan"
  line L0 (-24.9649, 136.9) -> (-24.6782, 141)
  line L1 (-24.6782, 141) -> (-41, 141)
  line L2 (-41, 141) -> (-41, 136.9)
  line L3 (-41, 136.9) -> (-24.9649, 136.9)
  dimension "d2322" = 24.9649
  dimension "d2323" = 136.9
  dimension "d2324" = 24.6782
  dimension "d2325" = 141
  dimension "d2326" = 41
  constraint horizontal L1
  constraint vertical L2
  constraint horizontal L3
  measures "d2322" horizontal distance of origin L0.start
  measures "d2323" vertical distance of origin L0.start
  measures "d2324" horizontal distance of origin L0.end
  measures "d2325" vertical distance of origin L0.end
  measures "d2326" horizontal distance of origin L1.end
extrude "R02 full width open front" cut sketch "草图17 (5)" along normal blind 154 bodies 1 in component "L1_DrainPan"
ref_plane "工作平面16" through (0, 0, 36) normal (0, 0, 1) x (1, 0, 0) in component "L1_RemovableGrate"
sketch "草图16 (6)" plane through (0, 0, 36) normal (0, 0, 1) x (1, 0, 0) in component "L1_RemovableGrate"
  line L0 (62.7, 59.7) -> (65.3, 59.7)
  line L1 (65.3, 59.7) -> (65.3, 65.3)
  line L2 (65.3, 65.3) -> (62.7, 65.3)
  line L3 (62.7, 65.3) -> (62.7, 59.7)
  dimension "d2332" = 59.7
  dimension "d2333" = 2.6
  dimension "d2334" = 5.6
  constraint horizontal L0
  constraint vertical L1
  constraint horizontal L2
  constraint vertical L3
  measures "d2332" vertical distance of origin L0.start
  measures "d2333" horizontal distance of L0.start L0.end
  measures "d2334" vertical distance of L0.end L1.end
extrude "R02 side locating notch 0" cut sketch "草图16 (6)" along normal blind 4 bodies 2 in component "L1_RemovableGrate"
ref_plane "工作平面18" through (0, 0, 20) normal (0, 0, 1) x (1, 0, 0) in component "L1_DrainPan"
sketch "草图18 (2)" plane through (0, 0, 20) normal (0, 0, 1) x (1, 0, 0) in component "L1_DrainPan"
  line L0 (63, 60) -> (65, 60)
  line L1 (65, 60) -> (65, 65)
  line L2 (65, 65) -> (63, 65)
  line L3 (63, 65) -> (63, 60)
  dimension "d2340" = 60
  dimension "d2341" = 2
  dimension "d2342" = 5
  constraint horizontal L0
  constraint vertical L1
  constraint horizontal L2
  constraint vertical L3
  measures "d2340" vertical distance of origin L0.start
  measures "d2341" horizontal distance of L0.start L0.end
  measures "d2342" vertical distance of L0.end L1.end
extrude "R02 side locating key 0" add sketch "草图18 (2)" along normal blind 20 bodies 1 in component "L1_DrainPan"
ref_plane "工作平面17" through (0, 0, 36) normal (0, 0, 1) x (1, 0, 0) in component "L1_RemovableGrate"
sketch "草图17 (6)" plane through (0, 0, 36) normal (0, 0, 1) x (1, 0, 0) in component "L1_RemovableGrate"
  line L0 (214.7, 59.7) -> (217.3, 59.7)
  line L1 (217.3, 59.7) -> (217.3, 65.3)
  line L2 (217.3, 65.3) -> (214.7, 65.3)
  line L3 (214.7, 65.3) -> (214.7, 59.7)
  dimension "d2347" = 214.7
  dimension "d2348" = 59.7
  dimension "d2349" = 2.6
  dimension "d2350" = 5.6
  constraint horizontal L0
  constraint vertical L1
  constraint horizontal L2
  constraint vertical L3
  measures "d2347" horizontal distance of origin L0.start
  measures "d2348" vertical distance of origin L0.start
  measures "d2349" horizontal distance of L0.start L0.end
  measures "d2350" vertical distance of L0.end L1.end
extrude "R02 side locating notch 1" cut sketch "草图17 (6)" along normal blind 4 bodies 2 in component "L1_RemovableGrate"
ref_plane "工作平面19" through (0, 0, 20) normal (0, 0, 1) x (1, 0, 0) in component "L1_DrainPan"
sketch "草图19 (2)" plane through (0, 0, 20) normal (0, 0, 1) x (1, 0, 0) in component "L1_DrainPan"
  line L0 (215, 60) -> (217, 60)
  line L1 (217, 60) -> (217, 65)
  line L2 (217, 65) -> (215, 65)
  line L3 (215, 65) -> (215, 60)
  dimension "d2355" = 215
  dimension "d2356" = 60
  dimension "d2357" = 2
  dimension "d2358" = 5
  constraint horizontal L0
  constraint vertical L1
  constraint horizontal L2
  constraint vertical L3
  measures "d2355" horizontal distance of origin L0.start
  measures "d2356" vertical distance of origin L0.start
  measures "d2357" horizontal distance of L0.start L0.end
  measures "d2358" vertical distance of L0.end L1.end
extrude "R02 side locating key 1" add sketch "草图19 (2)" along normal blind 20 bodies 1 in component "L1_DrainPan"
ref_plane "工作平面16" through (0, 0, 19.8) normal (0, 0, 1) x (1, 0, 0) in component "L2_Integrated"
sketch "草图16 (7)" plane through (0, 0, 19.8) normal (0, 0, 1) x (1, 0, 0) in component "L2_Integrated"
  line L0 (231, 140) -> (431, 140)
  line L1 (431, 140) -> (431, 167)
  line L2 (431, 167) -> (231, 167)
  line L3 (231, 167) -> (231, 140)
  dimension "d2363" = 231
  dimension "d2365" = 200
  dimension "d2366" = 27
  constraint horizontal L0
  constraint vertical L1
  constraint horizontal L2
  constraint vertical L3
  measures "d2363" horizontal distance of origin L0.start
  measures "d2365" horizontal distance of L0.start L0.end
  measures "d2366" vertical distance of L0.end L1.end
extrude "R02 remove projecting spout'" cut sketch "草图16 (7)" along normal blind 20.4 bodies 7 in component "L2_Integrated"
ref_plane "工作平面17" through (235, 0, 0) normal (1, 0, 0) x (0, 1, 0) in component "L2_Integrated"
sketch "草图17 (7)" plane through (235, 0, 0) normal (1, 0, 0) x (0, 0, -1) in component "L2_Integrated"
  line L0 (-24.9649, 136.9) -> (-24.6782, 141)
  line L1 (-24.6782, 141) -> (-41, 141)
  line L2 (-41, 141) -> (-41, 136.9)
  line L3 (-41, 136.9) -> (-24.9649, 136.9)
  dimension "d2371" = 24.9649
  dimension "d2372" = 136.9
  dimension "d2373" = 24.6782
  dimension "d2374" = 141
  dimension "d2375" = 41
  constraint horizontal L1
  constraint vertical L2
  constraint horizontal L3
  measures "d2371" horizontal distance of origin L0.start
  measures "d2372" vertical distance of origin L0.start
  measures "d2373" horizontal distance of origin L0.end
  measures "d2374" vertical distance of origin L0.end
  measures "d2375" horizontal distance of origin L1.end
extrude "R02 full width open front'" cut sketch "草图17 (7)" along normal blind 192 bodies 7 in component "L2_Integrated"
ref_plane "工作平面20" through (0, 0, 36) normal (0, 0, 1) x (1, 0, 0) in component "L2_RemovableGrate"
sketch "草图20" plane through (0, 0, 36) normal (0, 0, 1) x (1, 0, 0) in component "L2_RemovableGrate"
  line L0 (234.7, 59.7) -> (237.3, 59.7)
  line L1 (237.3, 59.7) -> (237.3, 65.3)
  line L2 (237.3, 65.3) -> (234.7, 65.3)
  line L3 (234.7, 65.3) -> (234.7, 59.7)
  dimension "d2381" = 59.7
  dimension "d2382" = 2.6
  dimension "d2383" = 5.6
  constraint horizontal L0
  constraint vertical L1
  constraint horizontal L2
  constraint vertical L3
  measures "d2381" vertical distance of origin L0.start
  measures "d2382" horizontal distance of L0.start L0.end
  measures "d2383" vertical distance of L0.end L1.end
extrude "R02 side locating notch 0'" cut sketch "草图20" along normal blind 4 bodies 8 in component "L2_RemovableGrate"
ref_plane "工作平面18" through (0, 0, 20) normal (0, 0, 1) x (1, 0, 0) in component "L2_Integrated"
sketch "草图18 (3)" plane through (0, 0, 20) normal (0, 0, 1) x (1, 0, 0) in component "L2_Integrated"
  line L0 (235, 60) -> (237, 60)
  line L1 (237, 60) -> (237, 65)
  line L2 (237, 65) -> (235, 65)
  line L3 (235, 65) -> (235, 60)
  dimension "d2389" = 60
  dimension "d2390" = 2
  dimension "d2391" = 5
  constraint horizontal L0
  constraint vertical L1
  constraint horizontal L2
  constraint vertical L3
  measures "d2389" vertical distance of origin L0.start
  measures "d2390" horizontal distance of L0.start L0.end
  measures "d2391" vertical distance of L0.end L1.end
extrude "R02 side locating key 0'" add sketch "草图18 (3)" along normal blind 20 bodies 7 in component "L2_Integrated"
ref_plane "工作平面21" through (0, 0, 36) normal (0, 0, 1) x (1, 0, 0) in component "L2_RemovableGrate"
sketch "草图21" plane through (0, 0, 36) normal (0, 0, 1) x (1, 0, 0) in component "L2_RemovableGrate"
  line L0 (424.7, 59.7) -> (427.3, 59.7)
  line L1 (427.3, 59.7) -> (427.3, 65.3)
  line L2 (427.3, 65.3) -> (424.7, 65.3)
  line L3 (424.7, 65.3) -> (424.7, 59.7)
  dimension "d2396" = 424.7
  dimension "d2397" = 59.7
  dimension "d2398" = 2.6
  dimension "d2399" = 5.6
  constraint horizontal L0
  constraint vertical L1
  constraint horizontal L2
  constraint vertical L3
  measures "d2396" horizontal distance of origin L0.start
  measures "d2397" vertical distance of origin L0.start
  measures "d2398" horizontal distance of L0.start L0.end
  measures "d2399" vertical distance of L0.end L1.end
extrude "R02 side locating notch 1'" cut sketch "草图21" along normal blind 4 bodies 8 in component "L2_RemovableGrate"
ref_plane "工作平面19" through (0, 0, 20) normal (0, 0, 1) x (1, 0, 0) in component "L2_Integrated"
sketch "草图19 (3)" plane through (0, 0, 20) normal (0, 0, 1) x (1, 0, 0) in component "L2_Integrated"
  line L0 (425, 60) -> (427, 60)
  line L1 (427, 60) -> (427, 65)
  line L2 (427, 65) -> (425, 65)
  line L3 (425, 65) -> (425, 60)
  dimension "d2404" = 425
  dimension "d2405" = 60
  dimension "d2406" = 2
  dimension "d2407" = 5
  constraint horizontal L0
  constraint vertical L1
  constraint horizontal L2
  constraint vertical L3
  measures "d2404" horizontal distance of origin L0.start
  measures "d2405" vertical distance of origin L0.start
  measures "d2406" horizontal distance of L0.start L0.end
  measures "d2407" vertical distance of L0.end L1.end
extrude "R02 side locating key 1'" add sketch "草图19 (3)" along normal blind 20 bodies 7 in component "L2_Integrated"
ref_plane "工作平面16" through (0, 0, 19.8) normal (0, 0, 1) x (1, 0, 0) in component "R1_Integrated"